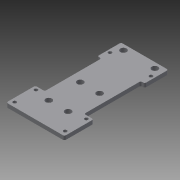
# Autodesk Inventor part: BottomSupport
Saved by Autodesk Inventor 2015 SP1 (Build 190203100, 203)
## iProperties
Created: 2015-09-23
Part Number: BottomSupport
Material: Generic
Document SubType Name: Modeling
Designer: I Rabey
Density: 1 g/cm^3
Appearance: Default
Author: I Rabey
Autodesk Inventor part; units mm, degrees
ref_plane "YZ Plane" through (0, 0, 0) normal (1, 0, 0) x (0, 1, 0)
ref_plane "XZ Plane" through (0, 0, 0) normal (0, 1, 0) x (-1, 0, 0)
ref_plane "XY Plane" through (0, 0, 0) normal (0, 0, 1) x (1, 0, 0)
sketch "Sketch2" plane through (0, 0, 0) normal (0, 1, 0) x (-1, 0, 0)
  line L0 (35, 0) -> (-35, 0)
  line L1 (-37, -2) -> (-37, -35)
  line L2 (-35, -37) -> (-27, -37)
  line L3 (-25, -39) -> (-25, -107)
  line L4 (-27, -109) -> (-28, -109)
  line L5 (-30, -111) -> (-30, -137)
  line L6 (-28, -139) -> (28, -139)
  line L7 (30, -137) -> (30, -111)
  line L8 (28, -109) -> (27, -109)
  line L9 (25, -107) -> (25, -39)
  line L10 (27, -37) -> (35, -37)
  line L11 (37, -35) -> (37, -2)
  circle A0 centre (19.95, -132) radius 3.95
  circle A1 centre (-19.95, -132) radius 3.95
  circle A2 centre (26, -121) radius 2.15
  circle A3 centre (-26, -121) radius 2.15
  circle A4 centre (12.319, -69.4) radius 3.95
  circle A5 centre (-12.321, -69.4) radius 3.95
  circle A6 centre (12.319, -29.4) radius 3.95
  circle A7 centre (-12.319, -29.4) radius 3.95
  circle A8 centre (32, -32.8) radius 2.15
  circle A9 centre (32, -5.8) radius 2.15
  circle A10 centre (-32, -33) radius 2.15
  circle A11 centre (-32, -6) radius 2.15
  arc A12 (25, -107) -> (27, -109) centre (27, -107) ccw
  arc A13 (30, -111) -> (28, -109) centre (28, -111) ccw
  arc A14 (27, -37) -> (25, -39) centre (27, -39) ccw
  arc A15 (35, -37) -> (37, -35) centre (35, -35) ccw
  arc A16 (37, -2) -> (35, 0) centre (35, -2) ccw
  arc A17 (-35, 0) -> (-37, -2) centre (-35, -2) ccw
  arc A18 (-37, -35) -> (-35, -37) centre (-35, -35) ccw
  arc A19 (-25, -39) -> (-27, -37) centre (-27, -39) ccw
  arc A20 (-27, -109) -> (-25, -107) centre (-27, -107) ccw
  arc A21 (-28, -109) -> (-30, -111) centre (-28, -111) ccw
  arc A22 (-30, -137) -> (-28, -139) centre (-28, -137) ccw
  arc A23 (28, -139) -> (30, -137) centre (28, -137) ccw
  point P0 (0, 0)
  point P1 (37, 0)
  point P2 (-37, 0)
  point P3 (-37, -37)
  point P4 (-25, -37)
  point P5 (-25, -109)
  point P6 (-30, -109)
  point P7 (-30, -139)
  point P8 (30, -139)
  point P9 (30, -109)
  point P10 (25, -109)
  point P11 (25, -37)
  point P12 (37, -37)
  dimension "d71" = 74
  dimension "d72" = 37
  dimension "d73" = 12
  dimension "d74" = 72
  dimension "d76" = 30
  dimension "d77" = 60
  dimension "d78" = 30
  dimension "d79" = 5
  dimension "d80" = 72
  dimension "d81" = 12
  dimension "d82" = 7.9
  dimension "d83" = 7.9
  dimension "d84" = 39.9
  dimension "d85" = 7
  dimension "d86" = 7
  dimension "d87" = 37
  dimension "d88" = 4.3
  dimension "d89" = 11
  dimension "d90" = 4
  dimension "d91" = 4.3
  dimension "d92" = 5
  dimension "d93" = 11
  dimension "d94" = 4
  dimension "d95" = 52
  dimension "d96" = 7.9
  dimension "d97" = 7.9
  dimension "d98" = 7.9
  dimension "d99" = 7.9
  dimension "d100" = 24.64
  dimension "d101" = 24.638
  dimension "d102" = 12.319
  dimension "d103" = 12.319
  dimension "d104" = 40
  dimension "d105" = 29.4
  dimension "d108" = 19.95
  dimension "d109" = 4.3
  dimension "d110" = 4.3
  dimension "d111" = 4.3
  dimension "d112" = 4.3
  dimension "d113" = 27
  dimension "d114" = 27
  dimension "d115" = 5
  dimension "d116" = 5
  dimension "d117" = 6
  dimension "d118" = 5.8
  dimension "d121" = 37
  dimension "d122" = 2
  dimension "d123" = 5
  dimension "d124" = 5
  dimension "d125" = 30
  constraints: 28 point on line, 24 centre point, 24 end point, 24 point on circle, 24 tangent, 11 equal radius, 6 perpendicular, 1 horizontal
  measures "d71" distance of point (37, 0) point (-37, 0)
  measures "d72" distance of point (-37, 0) point (-37, -37)
  measures "d73" distance of point (-37, -37) point (-25, -37)
  measures "d74" distance of point (-25, -37) point (-25, -109)
  measures "d76" distance of point (-30, -109) point (-30, -139)
  measures "d77" distance of point (-30, -139) point (30, -139)
  measures "d78" distance of point (30, -139) point (30, -109)
  measures "d79" distance of point (30, -109) point (25, -109)
  measures "d80" distance of point (25, -109) point (25, -37)
  measures "d81" distance of point (25, -37) point (37, -37)
  measures "d82" diameter of A0
  measures "d83" diameter of A1
  measures "d84" distance of A1.centre A0.centre
  measures "d85" distance from line of A1.centre L6
  measures "d86" distance from line of A0.centre L6
  measures "d87" distance from line of L11 point (0, 0)
  measures "d88" diameter of A2
  measures "d89" vertical distance of A0.centre A2.centre
  measures "d90" distance from line of A2.centre L7
  measures "d91" diameter of A3
  measures "d92" distance of point (-25, -109) point (-30, -109)
  measures "d93" vertical distance of A1.centre A3.centre
  measures "d94" distance from line of L5 A3.centre
  measures "d95" distance of A2.centre A3.centre
  measures "d96" diameter of A4
  measures "d97" diameter of A5
  measures "d98" diameter of A6
  measures "d99" diameter of A7
  measures "d100" distance of A5.centre A4.centre
  measures "d101" distance of A6.centre A7.centre
  measures "d102" horizontal distance of point (0, 0) A6.centre
  measures "d103" horizontal distance of point (0, 0) A4.centre
  measures "d104" distance of A6.centre A4.centre
  measures "d105" distance from line of L0 A6.centre
  measures "d108" horizontal distance of point (0, 0) A0.centre
  measures "d109" diameter of A8
  measures "d110" diameter of A9
  measures "d111" diameter of A10
  measures "d112" diameter of A11
  measures "d113" distance of A11.centre A10.centre
  measures "d114" distance of A8.centre A9.centre
  measures "d115" distance from line of L11 A9.centre
  measures "d116" distance from line of L1 A11.centre
  measures "d117" distance from line of L0 A11.centre
  measures "d118" distance from line of L0 A9.centre
  measures "d121" distance of point (37, -37) point (37, 0)
  measures "d122" radius of A12
  measures "d123" distance from line of L11 A8.centre
  measures "d124" distance from line of L1 A10.centre
  measures "d125" distance from line of point (0, 0) L7
extrude "Extrusion3" add sketch "Sketch2" along normal blind 5
equation "\"d72\" = d121"
equation "\"d78\" = d76"
body "Solid3"
